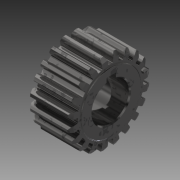
# Autodesk Inventor part: AM-0129 Small Final Gear 20T
Saved by Autodesk Inventor 2014 SP1 (Build 180222100, 222)
## iProperties
Shininess: 64.0
Length Units: 11272
Angle Units: 11279
Time Units: 11290
Mass Units: 11286
Length Display Precision: 3
Angle Display Precision: 2
Category: FIRST Robotics Components
Manager: Ed Sparks
Company: FIRST CAD Library
Created: 2003-12-13
Part Number: AM-0129 Small Final Gear 20T
Project: FIRST
Material: Steel, High Strength Low Alloy
Document SubType Name: Modeling
Designer: Ed Sparks
Engineer: Ed Sparks
Catalog Web Link: www.firstcadlibrary.com
Density: 7.84 g/cm^3
Mass: 40.2977 g
Surface Area: 36.6021 cm^2
Volume: 5.14001 cm^3
Appearance: Metal-Steel (Polished)
Density: 7.84
Volumn: 6.736982259993864
Area: 35.592573078640946
PropertySet Name: Model Information
Control State: 0
Master: False
Checked Out: False
Title: Gear
Subject: Robot Component
Author: Ed Sparks
Keywords: FIRST
Autodesk Inventor part; units mm, degrees
ref_plane "YZ Plane" through (0, 0, 0) normal (1, 0, 0) x (0, 1, 0)
ref_plane "XZ Plane" through (0, 0, 0) normal (0, 1, 0) x (-1, 0, 0)
ref_plane "XY Plane" through (0, 0, 0) normal (0, 0, 1) x (1, 0, 0)
sketch "Sketch2" plane through (7.112, 0, 0) normal (1, 0, 0) x (0, 0, -1)
  circle A0 centre (0, 0) radius 12.2955 construction
  arc A1 (1.7427, 13.8609) -> (-1.7427, 13.8609) centre (0, 0) ccw
  line L0 (0.9975, 12.6608) -> (4.004, 11.6253) construction
  line L1 (0, 0) -> (0, 25.7198) construction
  circle A2 centre (0, 0) radius 12.7 projected
  arc A3 (1.7427, 13.8609) -> (0.8342, 11.3719) centre (4.004, 11.6253) ccw
  arc A4 (-0.8342, 11.3719) -> (-1.7427, 13.8609) centre (-4.004, 11.6253) ccw
  arc A5 (0.5681, 11.098) -> (-0.5681, 11.098) centre (0, 0) ccw
  line L2 (0, 0) -> (0, 42.0936) construction
  circle A6 centre (0, 0) radius 6.35 projected
  circle A7 centre (0, 0) radius 12.7 construction
  line L3 (-4.004, 11.6253) -> (-0.9975, 12.6608) construction
  arc A8 (-0.8342, 11.3719) -> (-0.5681, 11.098) centre (-0.5811, 11.3516) ccw
  arc A9 (0.5681, 11.098) -> (0.8342, 11.3719) centre (0.5811, 11.3516) ccw
  dimension "d24" = 24.5909
  dimension "Root_Radius" = 11.1125
  dimension "d104" = 13.97
  dimension "Pitch_Diameter" = 25.4
  dimension "Tooth_Width" = 1.9949
  dimension "Root_Fillet" = 0.254
  dimension "d112" = 0.254
  constraints: 16 point on circle, 8 end point, 7 centre point, 6 coincident, 4 tangent, 1 point on line, 1 vertical, 6 other
  measures "Root_Radius" radius of A5
  measures "d104" radius of A1
  measures "Pitch_Diameter" diameter of A7
  measures "Tooth_Width" distance of L0.start L3.end
  measures "Root_Fillet" radius of A8
  measures "d112" radius of A9
sketch "Sketch1" plane through (0, 0, 0) normal (0, 0, 1) x (1, 0, 0)
  line L0 (7.112, 6.35) -> (7.112, 12.7)
  line L1 (6.3788, 13.97) -> (-6.3788, 13.97)
  line L2 (-7.112, 12.7) -> (-7.112, 6.35)
  line L3 (-7.112, 6.35) -> (7.112, 6.35)
  line L4 (7.112, 12.7) -> (6.3788, 13.97)
  line L5 (-7.112, 12.7) -> (-6.3788, 13.97)
  line L6 (-8.1229, 0) -> (10.8306, 0) projected
  line L7 (0, 0) -> (0, 27.4224) construction
  point P0 (0, 6.35)
  dimension "Bore_Radius" = 6.35
  dimension "Outside_Radius" = 13.97
  dimension "d77" = 12.7
  dimension "d108" = 30
  dimension "d109" = 30
  dimension "d110" = 14.224
  constraints: 14 end point, 3 vertical, 2 perpendicular, 1 coincident, 1 horizontal alignment, 1 midpoint, 1 point on line, 2 other
  measures "Bore_Radius" distance from line of point (0, 0) L3
  measures "Outside_Radius" distance from line of point (0, 0) L1
  measures "d77" distance from line of L6 L0.end
  measures "d108" angle of L5 L2
  measures "d109" angle of L4 L0
  measures "d110" distance of L2.end L0.start
revolve "Gear Blank" add sketch "Sketch1" angle 360 about axis through (-10, 0, 0) along (1, 0, 0)
extrude "Tooth Profile" cut sketch "Sketch2" against normal through all contours A3 A2 A4 A1 | A3 A9 A5 A8 A4 A2 picked at (0.0632, 12.1674)
pattern_circular "Circular Pattern" count 20 over 360 about axis through (0, 0, 0) along (1, 0, 0) of "Tooth Profile"
chamfer "Bore Chamfer Interior" [suppressed]
sketch "Sketch3" plane through (7.112, 11.6253, -4.004) normal (1, 0, 0) x (0, -0.1256275, -0.9920775)
  circle A0 centre (-2.5118, -12.0362) radius 6.35 projected
  arc A1 (5.9188, -0.0546) -> (3.9761, 0.4252) centre (-2.5118, -12.0362) ccw projected
  circle A2 centre (-2.5118, -12.0362) radius 10.16
  dimension "d31" = 20.32
  constraints: 1 centre point, 1 coincident, 1 other
  measures "d31" diameter of A2
extrude "Hub" add sketch "Sketch3" along normal blind 0.254
fillet "Hub Fillet" radius 0.254 2 edges at (7.112, 1.2764, 10.0795) (7.366, 1.2764, 10.0795)
chamfer "Bore Chamfer Exterior" distance 0.381 angle 45 1 edges at (-7.112, -6.35, 0)
chamfer "Bore Chamfer on Hub" distance 0.381 angle 45 1 edges at (7.366, 0.7977, 6.2997)
sketch "Sketch5" plane through (0, 0, 0) normal (1, 0, 0) x (0, 1, 0)
  line L0 (3.6662, 6.35) -> (7.3323, 0)
  line L1 (7.3323, 0) -> (3.6662, -6.35)
  line L2 (3.6662, -6.35) -> (-3.6662, -6.35)
  line L3 (-3.6662, -6.35) -> (-7.3323, 0)
  line L4 (-7.3323, 0) -> (-3.6662, 6.35)
  line L5 (-3.6662, 6.35) -> (3.6662, 6.35)
  point P0 (0, 0)
  dimension "d78" = 12.7
  constraints: 12 end point, 1 horizontal, 12 other
  measures "d78" distance between parallel lines of L1 L4
extrude "Hex Broach" [suppressed]
sketch "Sketch16" plane through (0, 0, 0) normal (1, 0, 0) x (0, 1, 0)
  line L0 (7.9375, -1.5875) -> (4.7625, -1.5875)
  line L1 (4.7625, -1.5875) -> (4.7625, 1.5875)
  line L2 (4.7625, 1.5875) -> (7.9375, 1.5875)
  line L3 (7.9375, 1.5875) -> (7.9375, -1.5875)
  line L4 (0, 0) -> (9.5781, 0) construction
  line L5 (0, 0) -> (0, 8.8774) construction
  dimension "d117" = 3.175
  dimension "d118" = 4.7625
  constraints: 12 end point, 3 horizontal, 2 parallel, 2 perpendicular, 2 vertical, 1 other
  measures "d117" distance of L2.end L0.start
  measures "d118" distance between parallel lines of L5 L1
extrude "Key" cut sketch "Sketch16" along normal through all both and the other way through all
equation "\"d31\" = Hub_Diameter"
equation "\"d32\" = Hub_Thickness"
equation "\"Bore_Radius\" = 0.5 * Bore"
equation "\"Bore\" = 12.7"
equation "\"Pressure_Angle\" = 14.5deg"
equation "\"Hub_Diameter\" = 20.32"
equation "\"Hub_Thickness\" = 0.254"
equation "\"Key_Size\" = 3.175"
equation "\"Bore_Chamfer\" = 0.381"
equation "\"Face_Width\" = 14.224"
equation "\"Tooth_Chamfer\" = 30deg"
body "Solid1"
